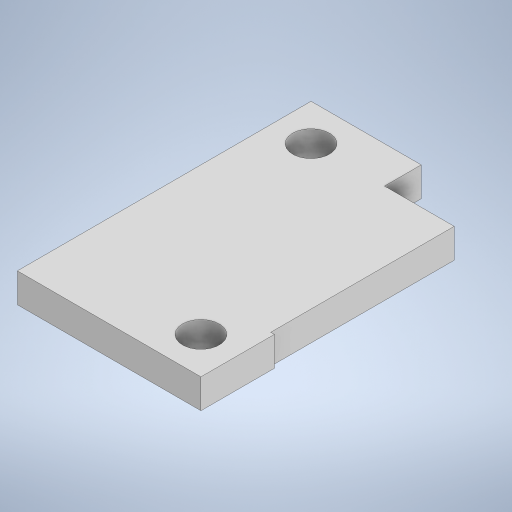
# Autodesk Inventor part: WPNA_TOP_MAINHOUSING
Saved by Autodesk Inventor 2024 (Build 280153000, 153)
## iProperties
Created: 2025-11-16
Part Number: WPNA_TOP_MAINHOUSING
Material: Generic
Document SubType Name: Modeling
Designer: albah
Density: 1 g/cm^3
Appearance: Default
Author: albah
Autodesk Inventor part; units mm, degrees
ref_plane "YZ Plane" through (0, 0, 0) normal (1, 0, 0) x (0, 1, 0)
ref_plane "XZ Plane" through (0, 0, 0) normal (0, 1, 0) x (-1, 0, 0)
ref_plane "XY Plane" through (0, 0, 0) normal (0, 0, 1) x (1, 0, 0)
sketch "Sketch1" plane through (0, 0, 0) normal (0, 1, 0) x (-1, 0, 0)
  line L0 (0, 0) -> (0, 70.5)
  line L1 (0, 70.5) -> (4.5, 70.5)
  circle A0 centre (4.5, 70.5) radius 2.5
  line L2 (0, 0) -> (0, 40.5)
  line L3 (0, 40.5) -> (19.5, 40.5)
  circle A1 centre (19.5, 40.5) radius 2.5
  line L4 (14.5, 45.5) -> (14.5, 35.5)
  line L5 (14.5, 35.5) -> (24.5, 35.5)
  line L6 (24.5, 35.5) -> (24.5, 45.5)
  line L7 (24.5, 45.5) -> (14.5, 45.5)
  line L8 (14.5, 45.5) -> (24.5, 35.5) construction
  line L9 (14.5, 35.5) -> (24.5, 45.5) construction
  line L10 (9.5, 75.5) -> (9.5, 65.5)
  line L11 (9.5, 65.5) -> (-0.5, 65.5)
  line L12 (-0.5, 65.5) -> (-0.5, 75.5)
  line L13 (-0.5, 75.5) -> (9.5, 75.5)
  line L14 (9.5, 75.5) -> (-0.5, 65.5) construction
  line L15 (9.5, 65.5) -> (-0.5, 75.5) construction
  line L16 (0, 0) -> (0, 42.5)
  line L17 (0, 42.5) -> (9.5, 42.5)
  line L18 (9.5, 42.5) -> (9.5, 35.5)
  line L19 (9.5, 35.5) -> (14.5, 35.5)
  line L20 (9.5, 75.5) -> (24.5, 75.5)
  line L21 (24.5, 75.5) -> (24.5, 45.5)
  point P0 (0, 65.5)
  point P1 (9.5, 40.5)
  dimension "d0" = 70.5
  dimension "d1" = 4.5
  dimension "d2" = 5
  dimension "d3" = 40.5
  dimension "d4" = 19.5
  dimension "d5" = 5
  dimension "d6" = 10
  dimension "d7" = 10
  dimension "d8" = 10
  dimension "d9" = 10
  dimension "d10" = 42.5
  dimension "d11" = 9.5
  constraints: 44 end point, 7 perpendicular, 4 midpoint, 4 parallel, 3 vertical, 2 centre point, 2 coincident, 2 horizontal, 2 point on line
  measures "d0" distance of L0.start L0.end
  measures "d1" distance of L0.end L1.end
  measures "d2" diameter of A0
  measures "d3" distance of L0.start L2.end
  measures "d4" distance of L2.end L3.end
  measures "d5" diameter of A1
  measures "d6" distance of L4.start L4.end
  measures "d7" distance of L5.end L4.end
  measures "d8" distance of L10.start L10.end
  measures "d9" distance of L10.end L11.end
  measures "d10" distance of L0.start L16.end
  measures "d11" distance of L16.end L17.end
extrude "Extrusion1" add sketch "Sketch1" along normal blind 4
body "Solid1"
